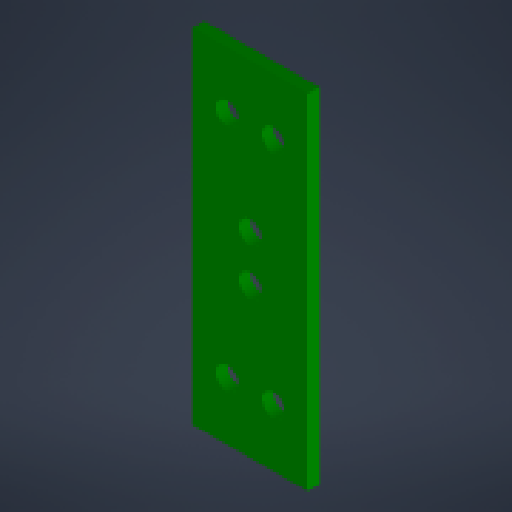
# Autodesk Inventor part: plate
Saved by Autodesk Inventor 2024 (Build 280153000, 153)
## iProperties
Created: 2023-04-17
Part Number: plate
Material: Типовые
Document SubType Name: Modeling
Designer: user
Density: 1 g/cm^3
Appearance: По умолчанию
Author: user
Autodesk Inventor part; units mm, degrees
ref_plane "YZ Plane" through (0, 0, 0) normal (1, 0, 0) x (0, 1, 0)
ref_plane "XZ Plane" through (0, 0, 0) normal (0, 1, 0) x (-1, 0, 0)
ref_plane "XY Plane" through (0, 0, 0) normal (0, 0, 1) x (1, 0, 0)
sketch "Эскиз2" plane through (0, 0, 0) normal (0, 1, 0) x (-1, 0, 0)
  line L0 (0, 0) -> (20, 0)
  line L1 (20, 0) -> (20, -60)
  line L2 (20, -60) -> (0, -60)
  line L3 (0, -60) -> (0, 0)
  dimension "d0" = 60
  dimension "d1" = 20
  constraints: 8 end point, 2 parallel, 1 horizontal, 1 perpendicular
  measures "d0" distance of L0.end L1.end
  measures "d1" distance of L1.end L2.end
extrude "Выдавливание1" add sketch "Эскиз2" along normal blind 2
sketch "Эскиз3" plane through (0, 2, 0) normal (0, 1, 0) x (1, 0, 0)
  circle A0 centre (-14, 10) radius 2 projected
  circle A1 centre (-6, 10) radius 2 projected
  circle A2 centre (-10, 26) radius 2 projected
  circle A3 centre (-10, 34) radius 2 projected
  circle A4 centre (-6, 50) radius 2 projected
  circle A5 centre (-14, 50) radius 2 projected
  point P0 (0, 0)
extrude "Выдавливание2" cut sketch "Эскиз3" against normal through all
